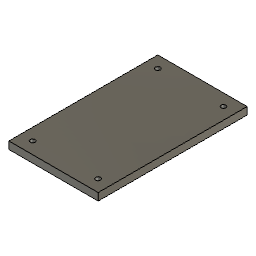
Mounting Plate (Autodesk Fusion 360 design; units mm, degrees)
part number: 2026-07-02-17-50-29-062
Autodesk Fusion 360 part; units mm, degrees
sketch "草图1" plane through (0, 0, 0) normal (0, 0, 1) x (1, 0, 0)
  line L0 (0, 0) -> (60, 0)
  line L1 (60, 0) -> (60, -100)
  line L2 (60, -100) -> (0, -100)
  line L3 (0, -100) -> (0, 0)
  dimension "d1" = 60
  dimension "d2" = 100
  constraint horizontal L0
  constraint vertical L1
  constraint horizontal L2
  constraint vertical L3
  constraint coincident L0.start L3.end
  measures "d1" distance of L0.start L0.end
  measures "d2" distance of L0.start L2.end
extrude "拉伸1" add sketch "草图1" along normal blind 5
sketch "草图2" plane through (0, 0, 5) normal (0, 0, 1) x (-1, 0, 0)
  line L0 (0, 100) -> (-60, 100)
  line L1 (-60, 100) -> (-60, 0)
  line L2 (-60, 0) -> (0, 0)
  line L3 (0, 0) -> (0, 100)
  circle A0 centre (-8, 8) radius 1.6
  circle A1 centre (-52, 8) radius 1.6
  circle A2 centre (-8, 92) radius 1.6
  circle A3 centre (-52, 92) radius 1.6
  dimension "d5" = 3.2
  dimension "d6" = 8
  dimension "d7" = 8
  dimension "d14" = -44
  dimension "d15" = 84
  measures "d5" diameter of A0
  measures "d6" distance of L3 A0.centre
  measures "d7" distance of L2 A0.centre
extrude "拉伸2" cut sketch "草图2" against normal blind 5 contours A0 | A1 | A2 | A3
